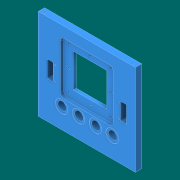
# Autodesk Inventor part: back
Saved by Autodesk Inventor 2016 SP1 (Build 200210100, 210)
## iProperties
Created: 2015-10-13
Part Number: back
Material: PC/ABS Plastic
Document SubType Name: Modeling
Designer: Sawaiz
Density: 0.357273 g/cm^3
Appearance: Cyan
Author: Sawaiz
Autodesk Inventor part; units mm, degrees
ref_plane "YZ Plane" through (0, 0, 0) normal (1, 0, 0) x (0, 1, 0)
ref_plane "XZ Plane" through (0, 0, 0) normal (0, 1, 0) x (-1, 0, 0)
ref_plane "XY Plane" through (0, 0, 0) normal (0, 0, 1) x (1, 0, 0)
sketch "Sketch1" plane through (0, 0, 0) normal (1, 0, 0) x (0, 1, 0)
  line L0 (-73.025, -68.2625) -> (73.025, -68.2625)
  line L1 (73.025, -68.2625) -> (73.025, 68.2625)
  line L2 (73.025, 68.2625) -> (-73.025, 68.2625)
  line L3 (-73.025, 68.2625) -> (-73.025, -68.2625)
  line L4 (-73.025, -68.2625) -> (73.025, 68.2625) construction
  line L5 (73.025, -68.2625) -> (-73.025, 68.2625) construction
  point P0 (0, 0)
  dimension "d0" = 146.05
  dimension "d1" = 136.525
  constraints: 12 end point, 2 midpoint, 2 parallel, 1 horizontal, 1 perpendicular
  measures "d0" distance of L2.end L1.end
  measures "d1" distance of L1.end L0.end
extrude "Extrusion1" add sketch "Sketch1" along normal blind 9.525
sketch "Sketch12" plane through (0, -73.025, 68.2625) normal (0, 0, 1) x (1, 0, 0)
  line L0 (0, 146.05) -> (9.525, 146.05) projected
  line L1 (0, 0) -> (9.525, 0) projected
  line L2 (0, 146.05) -> (0, 0) projected
  point P0 (0, 73.025)
  point P1 (6.35, 6.35)
  point P2 (6.35, 139.7)
  dimension "d131" = 6.35
  dimension "d139" = 6.35
  dimension "d140" = 6.35
  dimension "d141" = 6.35
  measures "d131" distance from line of L1 point (6.35, 6.35)
  measures "d139" distance from line of L2 point (6.35, 6.35)
  measures "d140" distance from line of L2 point (6.35, 139.7)
  measures "d141" distance from line of L0 point (6.35, 139.7)
hole "Hole6" at (6.35, -66.675, 68.2625) at (6.35, 66.675, 68.2625) direction (0, 0, -1) diameter 2.156 depth 8.865 tip angle 118 thread size "4-40 UNC" class "2B" standard "ANSI Unified Screw Threads"
sketch "Sketch15" plane through (0, 0, 0) normal (-1, 0, 0) x (0, 0, 1)
  circle A0 centre (-44.45, -44.45) radius 4.8514
  line L0 (-41.7048, -40.45) -> (-47.1952, -40.45)
  line L1 (-39.5986, -44.45) -> (-49.3014, -44.45)
  line L2 (-44.45, -44.45) -> (0, -44.45)
  line L3 (0, -44.45) -> (0, 0)
  line L4 (0, 0) -> (-44.45, 0)
  line L5 (-44.45, 0) -> (-44.45, -44.45)
  dimension "d162" = 9.7028
  dimension "d163" = 4
  dimension "d179" = 44.45
  dimension "d180" = 44.45
  constraints: 12 end point, 4 point on circle, 3 horizontal, 2 parallel, 1 centre point, 1 midpoint, 1 perpendicular
  measures "d162" diameter of A0
  measures "d163" distance between parallel lines of L0 L1
  measures "d179" distance of L2.end L3.end
  measures "d180" distance of L3.end L4.end
extrude "Extrusion8" [suppressed]
sketch "Sketch16" plane through (9.525, 0, 0) normal (1, 0, 0) x (0, 0, -1)
  arc A0 (41.7048, -40.45) -> (47.1952, -40.45) centre (44.45, -44.45) ccw projected
  point P0 (0, 0)
  constraints: 1 coincident
hole "Hole7" [suppressed]
sketch "Sketch17" plane through (9.525, 0, 0) normal (1, 0, 0) x (0, 0, -1)
  line L0 (68.2625, -73.025) -> (68.2625, 73.025) projected
  line L1 (68.2625, 73.025) -> (-68.2625, 73.025) projected
  line L2 (-68.2625, 73.025) -> (-68.2625, -73.025) projected
  line L3 (-68.2625, -73.025) -> (68.2625, -73.025) projected
  line L4 (-52.3875, -39.6875) -> (26.9875, -39.6875)
  line L5 (26.9875, -39.6875) -> (26.9875, 39.6875)
  line L6 (26.9875, 39.6875) -> (-52.3875, 39.6875)
  line L7 (-52.3875, 39.6875) -> (-52.3875, -39.6875)
  line L8 (-52.3875, -39.6875) -> (26.9875, 39.6875)
  line L9 (0, 0) -> (-68.2625, 0)
  point P0 (-12.7, 0)
  dimension "d174" = 79.375
  dimension "d175" = 79.375
  dimension "d176" = 12.7
  constraints: 12 end point, 2 midpoint, 2 parallel, 1 horizontal, 1 perpendicular, 1 point on line
  measures "d174" distance of L5.end L6.end
  measures "d175" distance of L4.end L5.end
  measures "d176" distance of point (-12.7, 0) L9.start
extrude "Extrusion9" cut sketch "Sketch17" against normal blind 4.7625 contours L8 L5 L4 | L7 L9 L8 | L7 L6 L8 L9
sketch "Sketch18" plane through (4.7625, 0, 0) normal (1, 0, 0) x (0, 0, -1)
  line L0 (-52.3875, -39.6875) -> (-52.3875, 39.6875) projected
  line L1 (26.9875, -39.6875) -> (-52.3875, -39.6875) projected
  line L2 (26.9875, 39.6875) -> (26.9875, -39.6875) projected
  line L3 (-52.3875, 39.6875) -> (26.9875, 39.6875) projected
  line L4 (-52.3875, -39.6875) -> (-52.3875, 39.6875) projected
  line L5 (-52.3875, -39.6875) -> (26.9875, 39.6875)
  line L6 (-38.1, -25.4) -> (12.7, -25.4)
  line L7 (12.7, -25.4) -> (12.7, 25.4)
  line L8 (12.7, 25.4) -> (-38.1, 25.4)
  line L9 (-38.1, 25.4) -> (-38.1, -25.4)
  line L10 (-38.1, -25.4) -> (12.7, 25.4) construction
  line L11 (12.7, -25.4) -> (-38.1, 25.4) construction
  point P0 (0, 0)
  point P1 (-12.7, 0)
  dimension "d181" = 50.8
  dimension "d182" = 50.8
  constraints: 14 end point, 3 midpoint, 2 parallel, 1 horizontal, 1 perpendicular
  measures "d181" distance of L8.end L7.end
  measures "d182" distance of L7.end L6.end
extrude "Extrusion10" cut sketch "Sketch18" against normal through all contours L9 L8 L5 | L5 L7 L6
fillet "Fillet3" radius 6.35 4 edges at (7.1438, -39.6875, -26.9875) (7.1438, -39.6875, 52.3875) (7.1438, 39.6875, 52.3875) (7.1438, 39.6875, -26.9875)
sketch "Sketch21" plane through (0, 0, 0) normal (-1, 0, 0) x (0, 0, 1)
  line L0 (-12.7, -25.4) -> (-12.7, 25.4) projected
  line L1 (-12.7, 25.4) -> (38.1, 25.4) projected
  line L2 (38.1, 25.4) -> (38.1, -25.4) projected
  line L3 (38.1, -25.4) -> (-12.7, -25.4) projected
  line L4 (-68.2625, -73.025) -> (-68.2625, 73.025) projected
  line L5 (68.2625, -73.025) -> (-68.2625, -73.025) projected
  line L6 (68.2625, 73.025) -> (68.2625, -73.025) projected
  line L7 (-68.2625, 73.025) -> (68.2625, 73.025) projected
  line L8 (-25.4, 38.1) -> (50.8, 38.1)
  line L9 (50.8, 38.1) -> (50.8, -38.1)
  line L10 (50.8, -38.1) -> (-25.4, -38.1)
  line L11 (-25.4, -38.1) -> (-25.4, 38.1)
  line L12 (-25.4, 38.1) -> (50.8, -38.1) construction
  line L13 (50.8, 38.1) -> (-25.4, -38.1) construction
  line L14 (0, 0) -> (12.7, 0)
  line L15 (44.45, -31.75) -> (44.45, 31.75)
  line L16 (44.45, 31.75) -> (-19.05, 31.75)
  line L17 (-19.05, 31.75) -> (-19.05, -31.75)
  line L18 (-19.05, -31.75) -> (44.45, -31.75)
  point P0 (44.45, 0)
  point P1 (12.7, -31.75)
  point P2 (-19.05, 0)
  point P3 (12.7, 31.75)
  dimension "d201" = 76.2
  dimension "d202" = 76.2
  dimension "d203" = 12.7
  dimension "d204" = 6.35
  constraints: 22 end point, 6 midpoint, 4 coincident, 4 parallel, 2 horizontal, 2 perpendicular, 3 other
  measures "d201" distance of L8.end L9.end
  measures "d202" distance of L9.end L10.end
  measures "d203" distance of L14.end L14.start
  measures "d204" distance between parallel lines of L9 L15
hole "Hole10" at (0, 31.75, 44.45) at (0, 0, 44.45) at (0, -31.75, 44.45) at (0, -31.75, 12.7) at (0, -31.75, -19.05) at (0, 0, -19.05) at (0, 31.75, -19.05) at (0, 31.75, 12.7) direction (1, 0, 0) diameter 3.264 end through all countersink diameter 5.715 countersink angle 82 clearance for "Flat Head Machine Screw (82)" size "#4" standard "Ansi Unified Screw Threads"
sketch "Sketch22" plane through (0, 0, 0) normal (-1, 0, 0) x (0, 0, 1)
  point P0 (0, 0)
  point P1 (-38.1, -12.7)
  dimension "d212" = 38.1
  dimension "d213" = 12.7
  measures "d212" horizontal distance of point (0, 0) point (-38.1, -12.7)
  measures "d213" vertical distance of point (0, 0) point (-38.1, -12.7)
hole "Hole11" at (0, -12.7, -38.1) direction (1, 0, 0) diameter 12.7 end through all
sketch "Sketch23" plane through (9.525, 0, 0) normal (1, 0, 0) x (0, 0, -1)
  circle A0 centre (38.1, -12.7) radius 6.35 projected
  point P0 (0, 0)
  constraints: 1 coincident
hole "Hole12" at (9.525, -12.7, -38.1) direction (-1, 0, 0) diameter 19.05 depth 0.8636
pattern_linear "Rectangular Pattern2" count 4 spacing 25.4 along (0, 1, 0) of "Hole11", "Hole12" first direction both ways yes
sketch "Sketch24" plane through (0, 0, 0) normal (-1, 0, 0) x (0, 0, 1)
  circle A0 centre (-38.1, 38.1) radius 6.35 projected
  circle A1 centre (-38.1, 12.7) radius 6.35 projected
  circle A2 centre (-38.1, -38.1) radius 6.35 projected
  circle A3 centre (-38.1, -12.7) radius 6.35 projected
  circle A4 centre (-19.05, 31.75) radius 2.8575 projected
  circle A5 centre (-19.05, -31.75) radius 2.8575 projected
  circle A6 centre (44.45, -31.75) radius 2.8575 projected
  circle A7 centre (44.45, 31.75) radius 2.8575 projected
  circle A8 centre (44.45, 0) radius 2.8575 projected
  circle A9 centre (12.7, -31.75) radius 2.8575 projected
  circle A10 centre (-19.05, 0) radius 2.8575 projected
  circle A11 centre (12.7, 31.75) radius 2.8575 projected
  line L0 (-12.7, -25.4) -> (-12.7, 25.4) projected
  line L1 (-12.7, 25.4) -> (38.1, 25.4) projected
  line L2 (38.1, 25.4) -> (38.1, -25.4) projected
  line L3 (38.1, -25.4) -> (-12.7, -25.4) projected
  line L4 (-68.2625, -73.025) -> (-68.2625, 73.025) projected
  line L5 (68.2625, -73.025) -> (-68.2625, -73.025) projected
  line L6 (68.2625, 73.025) -> (68.2625, -73.025) projected
  line L7 (-68.2625, 73.025) -> (68.2625, 73.025) projected
  line L8 (13.065, 59.5) -> (-13.065, 59.5)
  line L9 (-13.065, 59.5) -> (-13.065, 50.8)
  line L10 (-13.065, 50.8) -> (13.065, 50.8)
  line L11 (13.065, 50.8) -> (13.065, 59.5)
  line L12 (-13.065, 50.8) -> (13.065, 59.5) construction
  line L13 (-13.065, 59.5) -> (13.065, 50.8) construction
  line L14 (0, 55.15) -> (0, 0) construction
  dimension "d231" = 26.13
  dimension "d232" = 8.7
  dimension "d233" = 25.4
  constraints: 14 end point, 2 parallel, 1 horizontal, 1 midpoint, 1 perpendicular, 1 vertical
  measures "d231" distance of L9.end L10.end
  measures "d232" distance of L8.end L9.end
  measures "d233" distance between parallel lines of L1 L10
extrude "Extrusion11" cut sketch "Sketch24" against normal through all contours L11 L10 L9 L8
sketch "Sketch25" plane through (0, 0, 0) normal (-1, 0, 0) x (0, 0, 1)
  line L0 (-13.065, 50.8) -> (-13.065, 59.5) projected
  line L1 (-13.065, 59.5) -> (13.065, 59.5) projected
  line L2 (13.065, 59.5) -> (13.065, 50.8) projected
  line L3 (13.065, 50.8) -> (-13.065, 50.8) projected
  circle A0 centre (-38.1, 38.1) radius 6.35 projected
  circle A1 centre (-38.1, 12.7) radius 6.35 projected
  circle A2 centre (-38.1, -38.1) radius 6.35 projected
  circle A3 centre (-38.1, -12.7) radius 6.35 projected
  circle A4 centre (-19.05, 31.75) radius 2.8575 projected
  circle A5 centre (-19.05, -31.75) radius 2.8575 projected
  circle A6 centre (44.45, -31.75) radius 2.8575 projected
  circle A7 centre (44.45, 31.75) radius 2.8575 projected
  circle A8 centre (44.45, 0) radius 2.8575 projected
  circle A9 centre (12.7, -31.75) radius 2.8575 projected
  circle A10 centre (-19.05, 0) radius 2.8575 projected
  circle A11 centre (12.7, 31.75) radius 2.8575 projected
  line L4 (-12.7, -25.4) -> (-12.7, 25.4) projected
  line L5 (-12.7, 25.4) -> (38.1, 25.4) projected
  line L6 (38.1, 25.4) -> (38.1, -25.4) projected
  line L7 (38.1, -25.4) -> (-12.7, -25.4) projected
  line L8 (-68.2625, -73.025) -> (-68.2625, 73.025) projected
  line L9 (68.2625, -73.025) -> (-68.2625, -73.025) projected
  line L10 (68.2625, 73.025) -> (68.2625, -73.025) projected
  line L11 (-68.2625, 73.025) -> (68.2625, 73.025) projected
  line L12 (-10.715, 48.25) -> (10.715, 48.25) construction
  line L13 (-13.065, 50.8) -> (13.065, 50.8) projected
  line L14 (0, 50.8) -> (0, 48.25) construction
  point P0 (0, 0)
  dimension "d236" = 11.25
  dimension "d237" = 11.25
  dimension "d238" = 21.43
  constraints: 4 end point, 2 midpoint, 1 vertical
  measures "d236" distance from line of L12.end L1
  measures "d237" distance from line of L1 L12.start
  measures "d238" distance of L12.end L12.start
hole "Hole13" at (0, 48.25, 10.715) at (0, 48.25, -10.715) direction (1, 0, 0) diameter 2.3 end through all
mirror "Mirror2" about plane through (0, 0, 0) normal (0, 1, 0) of "Extrusion11", "Hole13"
fillet "Fillet4" radius 1 8 edges at (4.7625, -59.5, -13.065) (4.7625, -59.5, 13.065) (4.7625, -50.8, 13.065) (4.7625, -50.8, -13.065) (4.7625, 50.8, 13.065) (4.7625, 59.5, 13.065) (4.7625, 59.5, -13.065) (4.7625, 50.8, -13.065)
equation "\"height\" = 127"
equation "\"frameAcrylicThickness\" = 9.525"
equation "\"internalAcrylicThickness\" = 6.35"
equation "\"width\" = 127"
equation "\"depth\" = 273.05"
equation "\"mirrorAngle\" = 5deg"
equation "\"detectorWidth\" = 52"
equation "\"detectorHeight\" = 52"
equation "\"mirrorThickness\" = 3.175"
equation "\"fresnelThickness\" = 0.1"
equation "\"focalLength\" = 76.2"
equation "\"ior\" = 1.49"
equation "\"centerThickness\" = 1.524"
equation "\"fresnelAngle\" = 90deg"
equation "\"fresnelEffectiveDiameter\" = 152.4"
equation "\"oRingWidth\" = 1.5875"
equation "\"sensorHolderDepth\" = 19.05"
equation "\"aerogelClearence\" = 3.175"
equation "\"backplanePCBHeight\" = 76.2"
equation "\"backplanePCBWidth\" = 76.2"
equation "\"backplaneHoleOffsett\" = 6.35"
equation "\"backplanePostionOffsett\" = 12.7"
equation "\"moduleSlotClearence\" = 0.79375"
body "Solid1"
